Mast 2 (Autodesk Fusion 360 design; units mm, degrees)
Autodesk Fusion 360 part; units mm, degrees
sketch "Sketch1" plane through (0, 0, 0) normal (0, 0, 1) x (1, 0, 0)
  circle A0 centre (0, 0) radius 14.75
  circle A1 centre (0, 0) radius 11.75
  dimension "d1" = 29.5
  dimension "d2" = -3
  dimension "d3" = 23.5
  constraint coincident A0.centre A1.centre
  measures "d1" diameter of A0
  measures "d3" diameter of A1
  measures "d22" diameter of A0.centre
extrude "Extrude1" add sketch "Sketch1" along normal blind 70 makes body 1
sketch "Sketch3" plane through (0, 0, 70) normal (0, 0, 1) x (-1, 0, 0)
  circle A0 centre (0, 0) radius 11.75
  circle A1 centre (0, 0) radius 14.75
  circle A2 centre (0, 0) radius 14.75
  constraint coincident A0.centre A1.centre
ref_plane "WorkPlane1" through (0, 0, 78.4) normal (0, 0, 1) x (1, 0, 0)
sketch "Sketch2" plane through (0, 0, 78.4) normal (0, 0, 1) x (1, 0, 0)
  circle A0 centre (0, 0) radius 12.15
  circle A1 centre (0, 0) radius 14.75
  dimension "d7" = 24.3
  dimension "d8" = 29.5
  constraint coincident A0.centre A1.centre
  measures "d7" diameter of A0
  measures "d8" diameter of A1
loft "Loft1" add profiles "Sketch3", "Sketch2" section 1 section 2 contours A0 bodies 1
extrude "Extrude2" add sketch "Sketch2" along normal blind 7.4 contours A0 | A1 bodies 1
sketch "Sketch5" plane through (0, 0, 85.8) normal (0, 0, 1) x (-1, 0, 0)
  circle A0 centre (0, 0) radius 14.75
  circle A1 centre (0, 0) radius 14.75
  circle A2 centre (0, 0) radius 16.75
  dimension "d13" = 33.5
  constraint concentric A0 A1
  constraint coincident A0.centre A1.centre
  measures "d13" diameter of A2
extrude "Extrude3" add sketch "Sketch5" along normal blind 3.35 contours A0 A1 | A2 bodies 1
sketch "Sketch6" plane through (0, 0, 89.15) normal (0, 0, 1) x (-1, 0, 0)
  circle A0 centre (0, 0) radius 16.75
  circle A1 centre (0, 0) radius 16.75
  constraint coincident A0.centre A1.centre
ref_plane "WorkPlane2" through (0, 0, 92.05) normal (0, 0, 1) x (-1, 0, 0)
sketch "Sketch7" plane through (0, 0, 92.05) normal (0, 0, 1) x (1, 0, 0)
  circle A0 centre (0, 0) radius 13.75
  dimension "d16" = 27.5
  constraint coincident A0.centre origin
  measures "d16" diameter of A0
loft "Loft3" add profiles "Sketch7" section 1 face at (-0.9963, -4.3652, 89.15) section 2 on bodies 1 bodies 1
extrude "Extrude4" add 1 faces at (1.5859, 3.0843, 92.05) along direction (0, 0, 1) blind 7.7 on bodies 1 bodies 1
sketch "Sketch8" plane through (0, 0, 99.75) normal (0, 0, 1) x (-1, 0, 0)
  circle A0 centre (0, 0) radius 13.75
  circle A1 centre (0, 0) radius 31.9
  dimension "d19" = 63.8
  constraint coincident A0.centre A1.centre
  measures "d19" diameter of A1
extrude "Extrude5" add sketch "Sketch8" along normal blind 2 contours A0 | A1 bodies 1
sketch "Sketch9" plane through (0, 0, 101.75) normal (0, 0, 1) x (-1, 0, 0)
  circle A0 centre (0, 0) radius 31.9
  circle A1 centre (0, 0) radius 11.1
  circle A2 centre (0, 0) radius 7
  dimension "d22" = 22.2
  dimension "d27" = 14
  constraint concentric A0 A1
  constraint concentric A1 A2
  measures "d22" diameter of A1
  measures "d27" diameter of A2
extrude "Extrude6" cut sketch "Sketch9" against normal through all contours A2 bodies 1
extrude "Extrude7" cut sketch "Sketch9" against normal blind 7 contours A1 | A2 bodies 1
sketch "Sketch1 (2)" plane through (0, 0, 0) normal (0, 0, 1) x (1, 0, 0) in component "Mast_Foot"
  circle A0 centre (0, 0) radius 14.9
  circle A1 centre (0, 0) radius 20.9
  circle A2 centre (0, 0) radius 15.4
  dimension "d28" = 29.8
  dimension "d29" = 6
  dimension "d30" = 0.5
  constraint coincident A0.centre A1.centre
  measures "d28" diameter of A0
extrude "Extrude1'" add sketch "Sketch1 (2)" along normal blind 10 separate body contours A2 makes body 2 in component "Mast_Foot"
extrude "Extrude2'" add sketch "Sketch1 (2)" along normal blind 2 contours A1 bodies 2 in component "Mast_Foot"
sketch "Sketch2 (2)" plane through (0, 0, 0) normal (0, 1, 0) x (1, 0, 0) in component "Mast_Foot"
  line L0 (-15.4, -2) -> (15.4, -2)
  line L1 (-15.4, -10) -> (15.4, -10)
  line L2 (-20.9, -2) -> (20.9, -2)
  line L3 (15.4, -10) -> (15.4, -2)
  line L4 (20.9, -2) -> (15.4, -10)
  line L5 (15.4, -10) -> (13.4, -10)
  line L6 (13.4, -10) -> (13.4, -2)
  line L7 (13.4, -2) -> (15.4, -2)
  line L8 (15.4, -2) -> (15.4, -10)
  dimension "d35" = 2
  constraint coincident L1.end L3.start
  constraint coincident L0.end L3.end
  constraint coincident L2.end L4.start
  constraint horizontal L5
  constraint vertical L6
  constraint horizontal L7
  constraint vertical L8
  measures "d35" distance of L1.end L5.end
extrude "Extrude3'" add sketch "Sketch2 (2)" along normal mid plane 4 separate body makes body 3 in component "Mast_Foot"
extrude "Extrude4'" cut sketch "Sketch2 (2)" along normal mid plane 2 contours L2 L3 L4 L8 bodies 3 in component "Mast_Foot"
pattern_circular "C-Pattern1" count 8 over 360 about axis through (0, 0, 1.75) along (0, 0, 1) of bodies 3 makes body 4 at (13.1286, 10.3002, 4.6667) makes body 5 at (2, 16.5667, 4.6667) makes body 6 at (-13.1286, 10.3002, 4.6667) makes body 7 at (-16.5667, 2, 4.6667) makes body 8 at (-13.1286, -10.3002, 4.6667) makes body 9 at (-2, -16.5667, 4.6667) makes body 10 at (10.3002, -13.1286, 4.6667) in component "Mast_Foot"
extrude "Extrude5'" cut sketch "Sketch1 (2)" along normal through all contours A0 bodies 3 4 5 6 7 8 9 10 in component "Mast_Foot"
combine "Combine1" operation add target body 2 tool bodies 5 8 10 7 4 6 9 3 in component "Mast_Foot"
component "Mast_Foot" placed x (1, 0, 0) y (0, 1, 0) z (0, 0, 1) at (0, 0, 0)
named bodies: "Mast_Foot"
